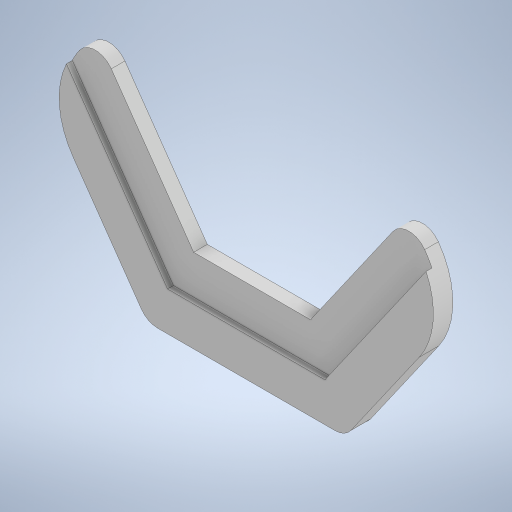
# Autodesk Inventor part: ДМС 045 держатель лотка
Saved by Autodesk Inventor 2024.2 (Build 282272000, 272)
## iProperties
Created: 2024-05-13
Part Number: ДМС 045 держатель лотка
Material: Generic
Document SubType Name: Modeling
Designer: admin
Density: 1 g/cm^3
Appearance: Default
Author: admin
Autodesk Inventor part; units mm, degrees
ref_plane "YZ Plane" through (0, 0, 0) normal (1, 0, 0) x (0, 1, 0)
ref_plane "XZ Plane" through (0, 0, 0) normal (0, 1, 0) x (-1, 0, 0)
ref_plane "XY Plane" through (0, 0, 0) normal (0, 0, 1) x (1, 0, 0)
sketch "Sketch1" plane through (0, 0, 0) normal (0, 1, 0) x (-1, 0, 0)
  line L0 (-30, 0) -> (30, 0)
  line L1 (-30, 0) -> (-79.0145, 70)
  line L2 (79.0145, 70) -> (30, 0)
  line L3 (88.8376, 14.2909) -> (50.8227, -40)
  line L4 (50.8227, -40) -> (-50.8227, -40)
  line L5 (-50.8227, -40) -> (-88.8376, 14.2909)
  line L6 (0, 0) -> (0, -40) construction
  arc A0 (88.8376, 14.2909) -> (79.0145, 70) centre (56.0715, 37.2339) ccw
  arc A1 (-79.0145, 70) -> (-88.8376, 14.2909) centre (-56.0715, 37.2339) ccw
  point P0 (0, 70)
  dimension "d1" = 60
  dimension "d3" = 40
  dimension "d5" = 40
  dimension "d16" = 125
  dimension "d17" = 70
  constraints: 14 end point, 4 point on circle, 2 centre point, 2 line through centre, 2 midpoint, 2 parallel, 2 tangent, 2 vertical alignment, 1 coincident, 1 equal length, 1 horizontal, 1 perpendicular, 1 other
  measures "d1" distance of L0.start L0.end
  measures "d3" distance between parallel lines of L4 L0
  measures "d5" distance between parallel lines of L3 L2
  measures "d16" angle of L0 L2
  measures "d17" distance from line of L0 L2.start
extrude "Extrusion1" add sketch "Sketch1" along normal blind 10
sketch "Sketch2" plane through (0, 0, 0) normal (0, -1, 0) x (1, 0, 0)
  line L0 (-30, 0) -> (30, 0) projected
  line L1 (-79.0145, 70) -> (-30, 0) projected
  line L2 (-50.8227, -40) -> (-88.8376, 14.2909) construction
  line L3 (50.8227, -40) -> (-50.8227, -40) construction
  line L4 (88.8376, 14.2909) -> (50.8227, -40) construction
  line L5 (30, 0) -> (79.0145, 70) projected
  line L6 (-92.3238, 54.1386) -> (-40.4113, -20)
  line L7 (-40.4113, -20) -> (40.4113, -20)
  line L8 (40.4113, -20) -> (92.3238, 54.1386)
  line L9 (-79.0145, 70) -> (-30, 0) projected
  line L10 (30, 0) -> (79.0145, 70) projected
  arc A0 (-79.0145, 70) -> (-88.8376, 14.2909) centre (-56.0715, 37.2339) ccw projected
  arc A1 (88.8376, 14.2909) -> (79.0145, 70) centre (56.0715, 37.2339) ccw projected
  point P0 (0, 0)
  dimension "d8" = 20
  dimension "d9" = 20
  dimension "d10" = 20
  constraints: 6 end point, 2 parallel, 2 point on circle, 1 horizontal
  measures "d8" distance between parallel lines of L7 L0
  measures "d9" distance between parallel lines of L1 L6
  measures "d10" distance between parallel lines of L5 L8
extrude "Extrusion2" cut sketch "Sketch2" against normal blind 3
fillet "Fillet1" radius 10 4 edges at (-79.0145, 6.5, 70) (79.0145, 6.5, 70) (-50.8227, 5, -40) (50.8227, 5, -40)
equation "\"d5\" = d3"
equation "\"d16\" = Лоток_угол"
equation "\"d9\" = d8"
equation "\"d10\" = d8"
equation "\"Лоток_угол\" = 125deg"
body "Solid1"
